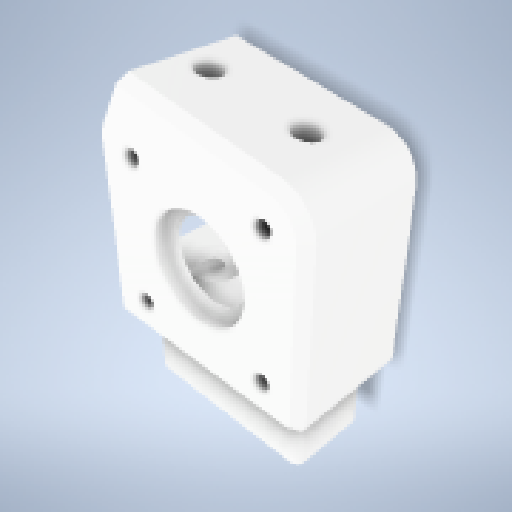
# Autodesk Inventor part: Y-axis Motor Block
Saved by Autodesk Inventor 2024 (Build 280153000, 153)
## iProperties
Created: 2024-08-08
Part Number: Y-axis Motor Block
Material: ABS Plastic
Document SubType Name: Modeling
Designer: Ishaan
Density: 1.06 g/cm^3
Appearance: Smooth - White
Author: Ishaan
Autodesk Inventor part; units mm, degrees
ref_plane "YZ Plane" through (0, 0, 0) normal (1, 0, 0) x (0, 1, 0)
sketch "Sketch1" plane through (0, 0, 0) normal (0, 0, 1) x (1, 0, 0)
  line L0 (24, -24) -> (-24, -24)
  line L1 (-24, -24) -> (-24, 24)
  line L2 (-24, 24) -> (24, 24)
  line L3 (24, 24) -> (24, -24)
  line L4 (24, -24) -> (-24, 24) construction
  line L5 (-24, -24) -> (24, 24) construction
  line L6 (-15.5, -15.5) -> (15.5, -15.5) construction
  line L7 (15.5, -15.5) -> (15.5, 15.5) construction
  line L8 (15.5, 15.5) -> (-15.5, 15.5) construction
  line L9 (-15.5, 15.5) -> (-15.5, -15.5) construction
  line L10 (-15.5, -15.5) -> (15.5, 15.5) construction
  line L11 (15.5, -15.5) -> (-15.5, 15.5) construction
  circle A0 centre (15.5, 15.5) radius 8.5
  line L12 (16.976, 23.8709) -> (-17.021, 29.8655)
  line L13 (-17.021, 29.8655) -> (-24, 17.7776)
  circle A1 centre (-15.5, 15.5) radius 8.5
  line L14 (-24, -24) -> (24, -24)
  point P0 (0, 0)
  point P1 (24, 15.5)
  point P2 (15.5, 24)
  point P3 (16.2437, 24)
  point P4 (-22.8612, 19.75)
  point P5 (-24, 15.5)
  point P6 (-20.4075, 24)
  dimension "d0" = 48
  dimension "d1" = 48
  dimension "d2" = 31
  dimension "d3" = 31
  dimension "d4" = 110
  dimension "d5" = 150
  constraints: 30 end point, 4 midpoint, 4 parallel, 3 horizontal, 2 coincident, 2 perpendicular, 2 tangent, 1 centre point, 1 point on line, 1 vertical, 4 other
  measures "d0" distance of L1.end L2.end
  measures "d1" distance of L0.end L1.end
  measures "d2" distance of L8.end L7.end
  measures "d3" distance of L7.end L6.end
  measures "d4" angle of L12 L13
  measures "d5" angle of L1 L13
extrude "Extrusion1" add sketch "Sketch1" along normal mid plane 28 contours L0 L1 A1 L2 A0 L3 | A0 | A1 | A0 L2 L12 | L2 L13 L12 | L13 L2 A1
sketch "Sketch2" plane through (0, 0, 14) normal (0, 0, 1) x (1, 0, 0)
  line L0 (15.5, -15.5) -> (-15.5, -15.5) construction
  line L1 (-15.5, -15.5) -> (-15.5, 15.5) construction
  line L2 (-15.5, 15.5) -> (15.5, 15.5) construction
  line L3 (15.5, 15.5) -> (15.5, -15.5) construction
  line L4 (15.5, -15.5) -> (-15.5, 15.5) construction
  line L5 (-15.5, -15.5) -> (15.5, 15.5) construction
  point P0 (0, 0)
  dimension "d8" = 31
  dimension "d9" = 31
  constraints: 12 end point, 4 coincident, 2 midpoint, 2 parallel, 1 horizontal, 1 perpendicular
  measures "d8" distance of L1.end L2.end
  measures "d9" distance of L0.end L1.end
hole "Hole1" at (-15.5, 15.5, 14) at (15.5, 15.5, 14) at (15.5, -15.5, 14) at (-15.5, -15.5, 14) direction (0, 0, -1) diameter 3.3 end through all
sketch "Sketch3" plane through (0, 0, -14) normal (0, 0, -1) x (-1, 0, 0)
  circle A0 centre (0, 0) radius 9
  dimension "d17" = 18
  constraints: 1 centre point, 1 coincident
  measures "d17" diameter of A0
extrude "Extrusion2" cut sketch "Sketch3" against normal through all
sketch "Sketch4" plane through (0, 0, 0) normal (0, 0, 1) x (1, 0, 0)
  circle A0 centre (0, 0) radius 9 projected
  circle A1 centre (-15.5, -15.5) radius 1.65 projected
  circle A2 centre (15.5, -15.5) radius 1.65 projected
  circle A3 centre (15.5, 15.5) radius 1.65 projected
  circle A4 centre (-15.5, 15.5) radius 1.65 projected
  line L0 (-22.8612, 19.75) -> (-17.021, 29.8655) projected
  line L1 (-17.021, 29.8655) -> (16.976, 23.8709) projected
  line L2 (0, 0) -> (-24, 0) construction
  line L3 (0, 11.5) -> (-24, 11.5)
  line L4 (-24, -11.5) -> (0, -11.5)
  arc A5 (0, -11.5) -> (0, 11.5) centre (0, 0) ccw
  arc A6 (-24, 11.5) -> (-24, -11.5) centre (-24, 0) ccw
  arc A7 (-22.8612, 19.75) -> (-24, 15.5) centre (-15.5, 15.5) ccw projected
  arc A8 (24, 15.5) -> (16.976, 23.8709) centre (15.5, 15.5) ccw projected
  line L5 (24, -24) -> (-24, -24) projected
  line L6 (-24, -24) -> (-24, 15.5) projected
  line L7 (24, 15.5) -> (24, -24) projected
  line L8 (-24, -24) -> (-24, 15.5) projected
  point P0 (-12, 0)
  dimension "d20" = 23
  constraints: 8 end point, 4 point on circle, 4 tangent, 2 centre point, 1 horizontal, 1 midpoint, 1 parallel, 1 point on line
  measures "d20" diameter of A6
ref_plane "Work Plane1" through (0, 0, -10.25) normal (0, 0, -1) x (-1, 0, 0)
ref_plane "Work Plane2" through (0, 0, 10.25) normal (0, 0, 1) x (1, 0, 0)
extrude "Extrusion4" cut sketch "Sketch4" against normal up to surface (20.5 mm away) from surface at 10.25 contours L6 A6 | L3 A5 L4 L6
fillet "Fillet1" radius 1 6 edges at (11.5, 0, -10.25) (-12, -11.5, -10.25) (-12, 11.5, -10.25) (11.5, 0, 10.25) (-12, -11.5, 10.25) (-12, 11.5, 10.25)
fillet "Fillet2" radius 1 8 edges at (-24, -11.2071, -9.9571) (-24, 0, -10.25) (-24, 11.2071, -9.9571) (-24, 11.5, 0) (-24, 11.2071, 9.9571) (-24, 0, 10.25) (-24, -11.2071, 9.9571) (-24, -11.5, 0)
chamfer "Chamfer1" distance 2 angle 45 1 edges at (9, 0, -14)
sketch "Sketch5" plane through (0, 0, 14) normal (0, 0, 1) x (1, 0, 0)
  circle A0 centre (0, 0) radius 11.25
  dimension "d32" = 22.5
  constraints: 1 centre point, 1 coincident
  measures "d32" diameter of A0
extrude "Extrusion5" cut sketch "Sketch5" against normal blind 2.5
fillet "Fillet8" radius 3 1 edges at (24, -24, 0)
chamfer "Chamfer3" distance 2 angle 45 10 edges at (-0.0225, 26.8682, -14) (22.0114, 20.9637, -14) (24, -2.75, -14) (23.1213, -23.1213, -14) (-1.5, -24, -14) (-0.0225, 26.8682, 14) (22.0114, 20.9637, 14) (24, -2.75, 14) (23.1213, -23.1213, 14) (-1.5, -24, 14)
sketch "Sketch6" plane through (0, 0, -14) normal (0, 0, -1) x (-1, 0, 0)
  circle A0 centre (0, 0) radius 11 projected
  circle A1 centre (15.5, -15.5) radius 1.65 projected
  circle A2 centre (-15.5, -15.5) radius 1.65 projected
  circle A3 centre (-15.5, 15.5) radius 1.65 projected
  circle A4 centre (15.5, 15.5) radius 1.65 projected
hole "Hole2" at (-15.5, -15.5, -14) at (15.5, -15.5, -14) at (-15.5, 15.5, -14) at (15.5, 15.5, -14) direction (0, 0, 1) diameter 6.5 depth 6.5
sketch "Sketch9" plane through (-24, -24, 12) normal (0, -1, 0) x (1, 0, 0)
  line L0 (4, -3) -> (44, -3)
  line L1 (44, -3) -> (44, -21)
  line L2 (44, -21) -> (4, -21)
  line L3 (4, -21) -> (4, -3)
  line L4 (4, -3) -> (44, -21) construction
  line L5 (44, -3) -> (4, -21) construction
  line L6 (0, -26) -> (45, -26) projected
  line L7 (0, -24) -> (0, 0) projected
  line L8 (24, -21.25) -> (24, -2.75) projected
  point P0 (24, -12)
  point P1 (24, -12)
  dimension "d73" = 18
  dimension "d74" = 40
  constraints: 12 end point, 3 midpoint, 2 parallel, 1 coincident, 1 horizontal, 1 perpendicular
  measures "d73" distance of L2.end L0.start
  measures "d74" distance of L1.end L2.end
extrude "Extrusion8" add sketch "Sketch9" along normal blind 14
sketch "Sketch10" plane through (-24, -38, 12) normal (0, -1, 0) x (1, 0, 0)
  line L0 (4, -21) -> (44, -21) construction
  line L1 (44, -21) -> (44, -3) construction
  line L2 (44, -3) -> (4, -3) construction
  line L3 (4, -3) -> (4, -21) construction
  point P0 (24, -12)
  point P1 (35, -12)
  point P2 (13, -12)
  point P3 (44, -12)
  dimension "d79" = 9
  dimension "d80" = 9
  dimension "d81" = 9
  dimension "d82" = 9
  dimension "d83" = 22
  constraints: 2 horizontal alignment, 1 midpoint
  measures "d79" distance from line of L1 point (35, -12)
  measures "d80" distance from line of L0 point (35, -12)
  measures "d81" distance from line of L0 point (13, -12)
  measures "d82" distance from line of L3 point (13, -12)
  measures "d83" distance of point (13, -12) point (35, -12)
hole "Hole4" at (-11, -38, 0) at (11, -38, 0) direction (0, 1, 0) diameter 5.3 depth 10
sketch "Sketch11" plane through (-11, -28, 0) normal (0, -1, 0) x (1, 0, 0)
  circle A0 centre (0, 0) radius 2.65 projected
  circle A1 centre (22, 0) radius 2.65 projected
  point P0 (11, 0)
hole "Hole5" at (-11, -28, 0) at (11, -28, 0) direction (0, 1, 0) diameter 10 depth 39.5
hole "Hole6" at (11, -28, 0) at (-11, -28, 0) direction (0, 1, 0) diameter 5 end through all
fillet "Fillet11" radius 2 4 edges at (20, -31, -9) (-20, -31, -9) (-20, -31, 9) (20, -31, 9)
fillet "Fillet12" radius 1 8 edges at (19.4142, -24, 8.4142) (20, -24, 0) (19.4142, -24, -8.4142) (0, -24, -9) (-19.4142, -24, -8.4142) (-20, -24, 0) (-19.4142, -24, 8.4142) (0, -24, 9)
fillet "Fillet13" radius 1 4 edges at (11.5, -0.0013, 4.9749) (11.5, 0, -4.9749) (11, 11.5, 5) (-11, -11.5, 5)
fillet "Fillet14" radius 1 2 edges at (-11, 28.8038, 2.5) (11, 24.9246, 2.5)
fillet "Fillet15" radius 0.5 4 edges at (-16, -17.0724, 0) (-16, -13.9276, -0.0024) (16, -17.0724, 0) (16, -13.9276, 0.0019)
equation "\"d79\" = d80"
equation "\"d82\" = d81"
body "Solid1"
